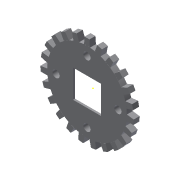
# Autodesk Inventor part: 200_Holder_Lambdaplate_1
Saved by Autodesk Inventor 2019 (Build 230136000, 136)
## iProperties
Created: 2019-07-08
Part Number: 200_Holder_Lambdaplate_1
Material: Generic
Document SubType Name: Modeling
Designer: diederichbenedict
Density: 1 g/cm^3
Appearance: Default
Author: diederichbenedict
Autodesk Inventor part; units mm, degrees
ref_plane "YZ Plane" through (0, 0, 0) normal (1, 0, 0) x (0, 1, 0)
ref_plane "XZ Plane" through (0, 0, 0) normal (0, 1, 0) x (-1, 0, 0)
ref_plane "XY Plane" through (0, 0, 0) normal (0, 0, 1) x (1, 0, 0)
sketch "Sketch1" plane through (0, 0, 0) normal (0, 0, 1) x (1, 0, 0)
  line L0 (5.25, 5.25) -> (-5.25, 5.25) projected
  line L1 (-5.25, 5.25) -> (-5.25, -5.25) projected
  line L2 (-5.25, -5.25) -> (5.25, -5.25) projected
  line L3 (5.25, -5.25) -> (5.25, 5.25) projected
  circle A0 centre (0, 0) radius 10
  line L4 (0, 0) -> (11.1419, 0)
  line L5 (0, 0) -> (11.515, -1.2103) construction
  line L6 (0, 0) -> (11.5784, 0) construction
  line L7 (0, 0) -> (11.515, 1.2103) construction
  line L8 (0, 0) -> (11.5784, 0) construction
  line L9 (-3.5, -3.5) -> (3.5, -3.5)
  line L10 (3.5, -3.5) -> (3.5, 3.5)
  line L11 (3.5, 3.5) -> (-3.5, 3.5)
  line L12 (-3.5, 3.5) -> (-3.5, -3.5)
  line L13 (-3.5, -3.5) -> (3.5, 3.5) construction
  line L14 (3.5, -3.5) -> (-3.5, 3.5) construction
  dimension "d0" = 20
  dimension "d1" = 6
  dimension "d2" = 6
  dimension "d3" = 7
  dimension "d4" = 7
  constraints: 22 end point, 4 horizontal, 2 equal length, 2 midpoint, 2 parallel, 1 centre point, 1 coincident, 1 perpendicular
  measures "d0" diameter of A0
  measures "d1" angle of L5 L6
  measures "d2" angle of L8 L7
  measures "d3" distance of L11.end L10.end
  measures "d4" distance of L10.end L9.end
extrude "Extrusion1" add sketch "Sketch1" along normal blind 0.5 contours L3 L2 L1 L0 | A0
sketch "Sketch2" plane through (0, 0, 0) normal (0, 0, -1) x (-1, 0, 0)
  line L0 (5.25, 5.25) -> (-5.25, 5.25) projected
  line L1 (-5.25, 5.25) -> (-5.25, -5.25) projected
  line L2 (-5.25, -5.25) -> (5.25, -5.25) projected
  line L3 (5.25, -5.25) -> (5.25, 5.25) projected
  circle A0 centre (0, 0) radius 10 projected
extrude "Extrusion2" add sketch "Sketch2" along normal blind 1
sketch "Sketch3" plane through (0, 0, -1) normal (0, 0, -1) x (-1, 0, 0)
  circle A0 centre (0, 0) radius 10 projected
  line L0 (7.7782, 0) -> (0, -7.7782) construction
  line L1 (0, -7.7782) -> (-7.7782, 0) construction
  line L2 (-7.7782, 0) -> (0, 7.7782) construction
  line L3 (0, 7.7782) -> (7.7782, 0) construction
  line L4 (7.7782, 0) -> (-7.7782, 0) construction
  line L5 (0, -7.7782) -> (0, 7.7782) construction
  line L6 (7.7782, 0) -> (18.7782, 0) construction
  dimension "d9" = 11
  dimension "d10" = 135
  dimension "d11" = 11
  constraints: 14 end point, 2 midpoint, 2 parallel, 1 equal length, 1 horizontal, 1 perpendicular
  measures "d9" distance of L0.start L0.end
  measures "d10" angle of L0 L6
  measures "d11" distance of L0.end L1.end
hole "Hole1" at (-7.7782, 0, -1) at (0, -7.7782, -1) at (7.7782, 0, -1) at (0, 7.7782, -1) direction (0, 0, 1) diameter 1.8 depth 16 tip angle 118
sketch "Sketch4" plane through (0, 0, 0.5) normal (0, 0, 1) x (1, 0, 0)
  line L0 (0, 0) -> (0.7457, 9.9737) construction
  line L1 (0, 0) -> (10.0015, 0) construction
  line L2 (0, 0) -> (0, 9.9909) construction
  line L3 (0, 0) -> (1.7838, 9.8396) construction
  circle A0 centre (0, 0) radius 10 construction
  line L4 (0, 0) -> (10, 0) construction
  line L5 (0.7457, 9.9737) -> (0.6289, 12)
  line L6 (0.6289, 12) -> (0, 12)
  line L7 (0, 12) -> (0, 9.9909)
  line L8 (0.6289, 12) -> (0, 0) construction
  circle A1 centre (0, 0) radius 10 construction
  arc A2 (0.7457, 9.9737) -> (0, 10) centre (-0.0309, -1.4483) ccw construction
  line L9 (-0.7457, 9.9737) -> (-0.6289, 12)
  line L10 (-0.6289, 12) -> (0, 12)
  arc A3 (0, 10) -> (-0.7457, 9.9737) centre (0.0309, -1.4483) ccw construction
  arc A4 (0.7457, 9.9737) -> (-0.7457, 9.9737) centre (0, -0.5734) ccw construction
  arc A5 (0.7457, 9.9737) -> (-0.7457, 9.9737) centre (0, -0.5734) ccw
  point P0 (-1.7838, 9.8396)
  dimension "d28" = 3
  dimension "d29" = 4.276
  dimension "d30" = 6
  dimension "d31" = 12
  constraints: 22 end point, 11 point on circle, 4 centre point, 4 symmetric about line, 3 horizontal, 2 equal length, 1 coincident, 1 collinear, 1 vertical, 3 other
  measures "d28" angle of L8 L2
  measures "d29" angle of L2 L0
  measures "d30" angle of L0 L3
  measures "d31" distance of point (0, 0) L6.end
extrude "Extrusion3" add sketch "Sketch4" against normal up to surface (1.5 mm away)
pattern_circular "Circular Pattern1" count 23 over 360 about axis through (0, 0, 0) along (0, 0, 1) of "Extrusion3"
sketch "Sketch5" plane through (0, 0, -1) normal (0, 0, -1) x (-1, 0, 0)
  point P0 (0, 0)
body "Solid1"
